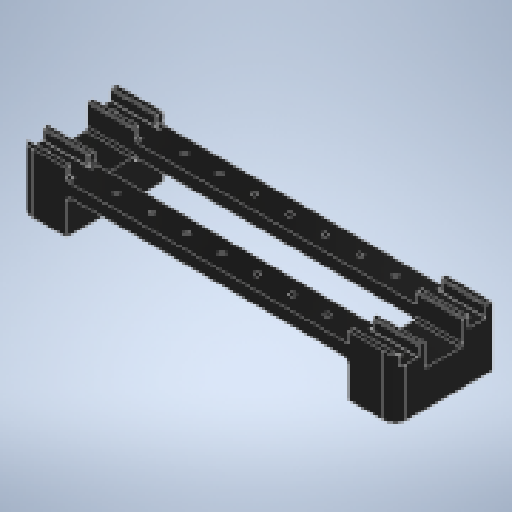
# Autodesk Inventor part: bridge_rails_support_ver2
Saved by Autodesk Inventor 2024 (Build 280153000, 153)
## iProperties
Created: 2025-06-26
Part Number: bridge_rails_support_ver2
Material: 一般
Document SubType Name: Modeling
Designer: kshau
Density: 1 g/cm^3
Appearance: 滑らか - 黒
Author: kshau
Autodesk Inventor part; units mm, degrees
ref_plane "YZ Plane" through (0, 0, 0) normal (1, 0, 0) x (0, 1, 0)
ref_plane "XZ Plane" through (0, 0, 0) normal (0, 1, 0) x (-1, 0, 0)
ref_plane "XY Plane" through (0, 0, 0) normal (0, 0, 1) x (1, 0, 0)
sketch "スケッチ1" plane through (0, 0, 0) normal (0, 0, 1) x (1, 0, 0)
  line L0 (0, 0) -> (20, 0)
  line L1 (20, 0) -> (20, 25.5)
  line L2 (20, 25.5) -> (0, 25.5)
  line L3 (0, 25.5) -> (0, 0)
  line L4 (20, 20.8) -> (140, 20.8)
  line L5 (140, 20.8) -> (140, 15.3)
  line L6 (140, 15.3) -> (20, 15.3)
  line L7 (20, 15.3) -> (20, 20.8)
  line L8 (140, 25.5) -> (160, 25.5)
  line L9 (160, 25.5) -> (160, 0)
  line L10 (160, 0) -> (140, 0)
  line L11 (140, 0) -> (140, 25.5)
  line L12 (160, 0) -> (20, 0)
  point P0 (20, 15.3)
  dimension "d0" = 25.5
  dimension "d1" = 20
  dimension "d3" = 5.5
  dimension "d4" = 120
  dimension "d6" = 20
  dimension "d61" = 4.7
  dimension "d62" = 4.7
  constraints: 26 end point, 6 parallel, 3 horizontal, 3 perpendicular, 2 point on line, 1 collinear
  measures "d0" distance of L2.end L0.start
  measures "d1" distance between parallel lines of L3 L1
  measures "d3" distance between parallel lines of L6 L4
  measures "d4" distance of L4.start L4.end
  measures "d6" distance of L8.start L8.end
  measures "d61" distance between parallel lines of L2 L4
  measures "d62" distance between parallel lines of L4 L8
extrude "押し出し1" add sketch "スケッチ1" along normal blind 41.5 contours L3 L2 L1 L0 | L1 L4 L5 L6 | L11 L5 L8 L9 L10
sketch "スケッチ2" plane through (140, 25.5, 0) normal (0, 1, 0) x (1, 0, 0)
  line L0 (-140, 0) -> (-140, -41.5) projected
  line L1 (20, 0) -> (20, -41.5) projected
  line L2 (-140, -29) -> (20, -29)
  line L3 (20, -29) -> (20, -12.5)
  line L4 (20, -12.5) -> (-140, -12.5)
  line L5 (-140, -12.5) -> (-140, -29)
  line L6 (20, -41.5) -> (0, -41.5) projected
  line L7 (20, 0) -> (0, 0) projected
  dimension "d10" = 12.5
  dimension "d11" = 12.5
  constraints: 8 end point, 2 parallel, 2 point on line, 1 horizontal, 1 perpendicular
  measures "d10" distance between parallel lines of L6 L2
  measures "d11" distance between parallel lines of L7 L4
extrude "押し出し2" cut sketch "スケッチ2" against normal blind 10.2
sketch "スケッチ3" plane through (140, 25.5, 41.5) normal (0, 1, 0) x (1, 0, 0)
  line L0 (-140, 41.5) -> (-140, 0) projected
  line L1 (-140, 2.6) -> (20, 2.6)
  line L2 (20, 12.5) -> (20, 0) projected
  line L3 (20, 0) -> (0, 0) projected
  line L4 (20, 9.9) -> (-140, 9.9)
  line L5 (-140, 38.9) -> (20, 38.9)
  line L6 (20, 41.5) -> (20, 0) projected
  line L7 (20, 31.6) -> (-140, 31.6)
  line L8 (-120, 41.5) -> (-140, 41.5) projected
  line L9 (20, 41.5) -> (0, 41.5) projected
  line L10 (0.3, 0) -> (0.3, 41.5)
  line L11 (-120, 0) -> (-140, 0) projected
  line L12 (-120.3, 0) -> (-120.3, 41.5)
  line L13 (0, 0) -> (-120, 0) projected
  line L14 (-120, 41.5) -> (-120, 0) projected
  line L15 (-120, 0) -> (-120, 41.5)
  line L16 (0, 41.5) -> (-120, 41.5) projected
  line L17 (0, 41.5) -> (0, 0)
  point P0 (15, 26.15)
  point P1 (-120.3, 2.6)
  point P2 (-120.3, 9.9)
  point P3 (-120.3, 31.6)
  point P4 (-120.3, 38.9)
  point P5 (0.3, 38.9)
  point P6 (0.3, 31.6)
  point P7 (0.3, 9.9)
  point P8 (0.3, 2.6)
  point P9 (0, 38.9)
  point P10 (-120, 38.9)
  point P11 (-120, 2.6)
  point P12 (0, 2.6)
  point P13 (0, 9.9)
  point P14 (-120, 9.9)
  point P15 (-120, 31.6)
  point P16 (0, 31.6)
  dimension "d14" = 2.6
  dimension "d15" = 7.3
  dimension "d16" = 2.6
  dimension "d17" = 7.3
  dimension "d38" = 19.7
  dimension "d39" = 19.7
  constraints: 16 end point, 12 point on line, 5 perpendicular, 2 horizontal, 1 parallel
  measures "d14" distance between parallel lines of L3 L1
  measures "d15" distance between parallel lines of L1 L4
  measures "d16" distance between parallel lines of L8 L5
  measures "d17" distance between parallel lines of L5 L7
  measures "d38" distance between parallel lines of L6 L10
  measures "d39" distance between parallel lines of L0 L12
extrude "押し出し3" cut sketch "スケッチ3" against normal blind 4.7 contours L5 L12 L7 L0 | L8 L14 L5 L12 | L5 L14 L7 L12 | L4 L12 L1 L0 | L7 L14 L4 L12 | L5 L17 L7 L14 | L9 L10 L5 L17 | L4 L14 L1 L12 | L5 L10 L7 L17 | L1 L14 L11 L12 | L4 L17 L1 L14 | L7 L10 L4 L17 | L5 L6 L7 L10 | L4 L10 L1 L17 | L1 L10 L3 L17 | L4 L2 L1 L10
fillet "フィレット1" radius 5 2 edges at (160, 12.75, 41.5) (0, 12.75, 41.5)
sketch "スケッチ4" plane through (20, 20.8, 0) normal (0, 1, 0) x (1, 0, 0)
  line L0 (140, -2.6) -> (140, -9.9) projected
  line L1 (140, -6.25) -> (-20, -6.25)
  line L2 (-20, -9.9) -> (-20, -2.6) projected
  line L3 (-0.3, -38.9) -> (-19.3863, -38.9) projected
  line L4 (120.3, -31.6) -> (140, -31.6) projected
  line L5 (139.4, -35.25) -> (-20, -35.25)
  line L6 (-20, 0) -> (-20, -36.5) projected
  line L7 (-20, -31.6) -> (-0.3, -31.6) projected
  line L8 (140, -31.6) -> (140, -36.5) projected
  point P0 (135, -6.25)
  point P1 (139.3863, -38.9)
  point P2 (135, -35.25)
  point P3 (120, -35.25)
  point P4 (120, -6.25)
  point P5 (105, -35.25)
  point P6 (105, -6.25)
  point P7 (90, -35.25)
  point P8 (90, -6.25)
  point P9 (75, -35.25)
  point P10 (75, -6.25)
  point P11 (60, -35.25)
  point P12 (60, -6.25)
  point P13 (45, -35.25)
  point P14 (45, -6.25)
  point P15 (30, -35.25)
  point P16 (30, -6.25)
  point P17 (15, -35.25)
  point P18 (15, -6.25)
  point P19 (0, -35.25)
  point P20 (0, -6.25)
  point P21 (-15, -35.25)
  point P22 (-15, -6.25)
  dimension "d21" = 5
  dimension "d22" = 3.65
  dimension "d23" = 5
  dimension "d26" = 15
  constraints: 4 end point, 3 point on line, 2 horizontal, 2 midpoint, 21 other
  measures "d21" distance from line of L0 point (135, -6.25)
  measures "d22" distance between parallel lines of L7 L5
  measures "d26" distance of point (135, -35.25) point (120, -35.25)
hole "穴1" at (155, 20.8, 35.25) at (125, 20.8, 35.25) at (110, 20.8, 35.25) at (95, 20.8, 35.25) at (80, 20.8, 35.25) at (65, 20.8, 35.25) at (50, 20.8, 35.25) at (35, 20.8, 35.25) at (5, 20.8, 35.25) at (35, 20.8, 6.25) at (5, 20.8, 6.25) at (50, 20.8, 6.25) at (65, 20.8, 6.25) at (80, 20.8, 6.25) at (95, 20.8, 6.25) at (110, 20.8, 6.25) at (125, 20.8, 6.25) at (155, 20.8, 6.25) direction (0, -1, 0) diameter 2.3 end through all
sketch "スケッチ5" plane through (20, 15.3, 41.5) normal (0, -1, 0) x (1, 0, 0)
  circle A0 centre (15, -6.25) radius 1.15 projected
  circle A1 centre (15, -6.25) radius 2.5403
  line L0 (15, -6.25) -> (15, -3.7097)
  line L1 (13.7298, -4.05) -> (16.2702, -4.05)
  line L2 (16.2702, -4.05) -> (15, -6.25)
  line L3 (12.4597, -6.25) -> (13.7298, -4.05)
  line L4 (13.7298, -8.45) -> (12.4597, -6.25)
  line L5 (16.2702, -8.45) -> (13.7298, -8.45)
  line L6 (17.5403, -6.25) -> (16.2702, -8.45)
  line L7 (16.2702, -4.05) -> (17.5403, -6.25)
  circle A2 centre (15, -35.25) radius 1.15 projected
  circle A3 centre (15, -35.25) radius 2.5403
  line L8 (15, -35.25) -> (15, -32.7097)
  line L9 (16.2702, -33.05) -> (15, -35.25)
  line L10 (16.2702, -33.05) -> (13.7298, -33.05)
  line L11 (13.7298, -33.05) -> (12.4597, -35.25)
  line L12 (12.4597, -35.25) -> (13.7298, -37.45)
  line L13 (13.7298, -37.45) -> (16.2702, -37.45)
  line L14 (16.2702, -37.45) -> (17.5403, -35.25)
  line L15 (17.5403, -35.25) -> (16.2702, -33.05)
  line L16 (0, -41.5) -> (0, -12.5) projected
  line L17 (0, -41.5) -> (120, -41.5) projected
  line L18 (0, -41.5) -> (120, -41.5)
  line L19 (27.4597, -35.25) -> (28.7298, -37.45)
  line L20 (28.7298, -33.05) -> (27.4597, -35.25)
  line L21 (31.2702, -33.05) -> (28.7298, -33.05)
  line L22 (32.5403, -35.25) -> (31.2702, -33.05)
  line L23 (31.2702, -37.45) -> (32.5403, -35.25)
  line L24 (28.7298, -37.45) -> (31.2702, -37.45)
  line L25 (28.7298, -4.05) -> (31.2702, -4.05)
  line L26 (27.4597, -6.25) -> (28.7298, -4.05)
  line L27 (28.7298, -8.45) -> (27.4597, -6.25)
  line L28 (31.2702, -8.45) -> (28.7298, -8.45)
  line L29 (32.5403, -6.25) -> (31.2702, -8.45)
  line L30 (31.2702, -4.05) -> (32.5403, -6.25)
  line L31 (42.4597, -35.25) -> (43.7298, -37.45)
  line L32 (43.7298, -33.05) -> (42.4597, -35.25)
  line L33 (46.2702, -33.05) -> (43.7298, -33.05)
  line L34 (47.5403, -35.25) -> (46.2702, -33.05)
  line L35 (46.2702, -37.45) -> (47.5403, -35.25)
  line L36 (43.7298, -37.45) -> (46.2702, -37.45)
  line L37 (43.7298, -4.05) -> (46.2702, -4.05)
  line L38 (42.4597, -6.25) -> (43.7298, -4.05)
  line L39 (43.7298, -8.45) -> (42.4597, -6.25)
  line L40 (46.2702, -8.45) -> (43.7298, -8.45)
  line L41 (47.5403, -6.25) -> (46.2702, -8.45)
  line L42 (46.2702, -4.05) -> (47.5403, -6.25)
  line L43 (57.4597, -35.25) -> (58.7298, -37.45)
  line L44 (58.7298, -33.05) -> (57.4597, -35.25)
  line L45 (61.2702, -33.05) -> (58.7298, -33.05)
  line L46 (62.5403, -35.25) -> (61.2702, -33.05)
  line L47 (61.2702, -37.45) -> (62.5403, -35.25)
  line L48 (58.7298, -37.45) -> (61.2702, -37.45)
  line L49 (58.7298, -4.05) -> (61.2702, -4.05)
  line L50 (57.4597, -6.25) -> (58.7298, -4.05)
  line L51 (58.7298, -8.45) -> (57.4597, -6.25)
  line L52 (61.2702, -8.45) -> (58.7298, -8.45)
  line L53 (62.5403, -6.25) -> (61.2702, -8.45)
  line L54 (61.2702, -4.05) -> (62.5403, -6.25)
  line L55 (72.4597, -35.25) -> (73.7298, -37.45)
  line L56 (73.7298, -33.05) -> (72.4597, -35.25)
  line L57 (76.2702, -33.05) -> (73.7298, -33.05)
  line L58 (77.5403, -35.25) -> (76.2702, -33.05)
  line L59 (76.2702, -37.45) -> (77.5403, -35.25)
  line L60 (73.7298, -37.45) -> (76.2702, -37.45)
  line L61 (73.7298, -4.05) -> (76.2702, -4.05)
  line L62 (72.4597, -6.25) -> (73.7298, -4.05)
  line L63 (73.7298, -8.45) -> (72.4597, -6.25)
  line L64 (76.2702, -8.45) -> (73.7298, -8.45)
  line L65 (77.5403, -6.25) -> (76.2702, -8.45)
  line L66 (76.2702, -4.05) -> (77.5403, -6.25)
  line L67 (87.4597, -35.25) -> (88.7298, -37.45)
  line L68 (88.7298, -33.05) -> (87.4597, -35.25)
  line L69 (91.2702, -33.05) -> (88.7298, -33.05)
  line L70 (92.5403, -35.25) -> (91.2702, -33.05)
  line L71 (91.2702, -37.45) -> (92.5403, -35.25)
  line L72 (88.7298, -37.45) -> (91.2702, -37.45)
  line L73 (88.7298, -4.05) -> (91.2702, -4.05)
  line L74 (87.4597, -6.25) -> (88.7298, -4.05)
  line L75 (88.7298, -8.45) -> (87.4597, -6.25)
  line L76 (91.2702, -8.45) -> (88.7298, -8.45)
  line L77 (92.5403, -6.25) -> (91.2702, -8.45)
  line L78 (91.2702, -4.05) -> (92.5403, -6.25)
  line L79 (102.4597, -35.25) -> (103.7298, -37.45)
  line L80 (103.7298, -33.05) -> (102.4597, -35.25)
  line L81 (106.2702, -33.05) -> (103.7298, -33.05)
  line L82 (107.5403, -35.25) -> (106.2702, -33.05)
  line L83 (106.2702, -37.45) -> (107.5403, -35.25)
  line L84 (103.7298, -37.45) -> (106.2702, -37.45)
  line L85 (103.7298, -4.05) -> (106.2702, -4.05)
  line L86 (102.4597, -6.25) -> (103.7298, -4.05)
  line L87 (103.7298, -8.45) -> (102.4597, -6.25)
  line L88 (106.2702, -8.45) -> (103.7298, -8.45)
  line L89 (107.5403, -6.25) -> (106.2702, -8.45)
  line L90 (106.2702, -4.05) -> (107.5403, -6.25)
  point P0 (-20, -41.5)
  point P1 (0, -29)
  point P2 (102.4597, -6.25)
  point P3 (107.5403, -6.25)
  point P4 (87.4597, -6.25)
  point P5 (92.5403, -6.25)
  point P6 (72.4597, -35.25)
  point P7 (77.5403, -35.25)
  point P8 (72.4597, -6.25)
  point P9 (77.5403, -6.25)
  point P10 (57.4597, -6.25)
  point P11 (62.5403, -6.25)
  point P12 (42.4597, -6.25)
  point P13 (47.5403, -6.25)
  point P14 (57.4597, -35.25)
  point P15 (42.4597, -35.25)
  point P16 (27.4597, -35.25)
  point P17 (32.5403, -35.25)
  point P18 (12.4597, -35.25)
  point P19 (13.7298, -37.45)
  point P20 (27.4597, -6.25)
  point P21 (28.7298, -8.45)
  point P22 (31.2702, -8.45)
  point P23 (32.5403, -6.25)
  point P24 (13.7298, -4.05)
  point P25 (12.4597, -6.25)
  point P26 (13.7298, -8.45)
  point P27 (16.2702, -8.45)
  point P28 (17.5403, -6.25)
  dimension "d40" = 2.2
  dimension "d41" = 30
  dimension "d44" = 360
  dimension "d46" = 30
  dimension "d47" = 2.2
  dimension "d50" = 360
  dimension "d54" = 15
  constraints: 178 end point, 6 point on circle, 2 centre point, 2 coincident, 2 collinear, 2 perpendicular, 2 vertical, 1 horizontal, 253 other
  measures "d40" distance from line of A1.centre L1
  measures "d41" angle of L0 L2
  measures "d46" angle of L8 L9
  measures "d47" distance from line of L8.start L10
  measures "d54" distance of L12.start L19.start
extrude "押し出し4" cut sketch "スケッチ5" against normal blind 2 contours A0 L2 L7 L6 L5 L4 L3 L1 L0 | A0 L0 L1 L2 | A2 L9 L15 L14 L13 L12 L11 L10 L8 | A2 L8 L10 L9 | L20 L21 L22 L23 L24 L19 | L25 L30 L29 L28 L27 L26 | L32 L33 L34 L35 L36 L31 | L37 L42 L41 L40 L39 L38 | L44 L45 L46 L47 L48 L43 | L49 L54 L53 L52 L51 L50 | L56 L57 L58 L59 L60 L55 | L61 L66 L65 L64 L63 L62 | L68 L69 L70 L71 L72 L67 | L73 L78 L77 L76 L75 L74 | L80 L81 L82 L83 L84 L79 | L85 L90 L89 L88 L87 L86
fillet "フィレット2" radius 0.1 8 edges at (9.85, 20.8, 31.6) (10.1568, 20.8, 38.9) (9.85, 20.8, 2.6) (9.85, 20.8, 9.9) (150.15, 20.8, 2.6) (150.15, 20.8, 9.9) (150.15, 20.8, 31.6) (149.8432, 20.8, 38.9)
fillet "フィレット3" radius 1 20 edges at (150, 15.3, 12.5) (150, 15.3, 29) (140.3, 20.8, 38.85) (140.3, 20.8, 40.2) (140.3, 20.8, 31.65) (140.3, 20.8, 30.3) (140.3, 20.8, 1.3) (140.3, 20.8, 11.2) (140.3, 20.8, 2.65) (140.3, 20.8, 9.85) (10, 15.3, 12.5) (10, 15.3, 29) (19.7, 20.8, 40.2) (19.7, 20.8, 38.85) (19.7, 20.8, 30.3) (19.7, 20.8, 31.65) (19.7, 20.8, 2.65) (19.7, 20.8, 9.85) (19.7, 20.8, 1.3) (19.7, 20.8, 11.2)
fillet "フィレット4" radius 0.5 28 edges at (9.85, 25.5, 2.6) (9.85, 25.5, 9.9) (9.85, 25.5, 31.6) (10.1568, 25.5, 38.9) (150.15, 25.5, 2.6) (150.15, 25.5, 9.9) (150.15, 25.5, 29) (149.8432, 25.5, 38.9) (139.5236, 20.8253, 2.6) (20.4764, 20.8253, 2.6) (140.3, 23.65, 2.6) (139.5236, 20.8253, 9.9) (140.3, 23.65, 9.9) (150.15, 25.5, 31.6) (150.15, 25.5, 12.5) (139.5236, 20.8253, 38.9) (20.4764, 20.8253, 38.9) (140.3, 23.65, 38.9) (20.4764, 20.8253, 31.6) (139.5236, 20.8253, 31.6) (140.3, 23.65, 31.6) (9.85, 25.5, 12.5) (9.85, 25.5, 29) (19.7, 23.65, 2.6) (20.4764, 20.8253, 9.9) (19.7, 23.65, 9.9) (19.7, 23.65, 31.6) (19.7, 23.65, 38.9)
fillet "フィレット5" radius 2 4 edges at (20, 15.3, 35.25) (20, 15.3, 6.25) (140, 15.3, 35.25) (140, 15.3, 6.25)
